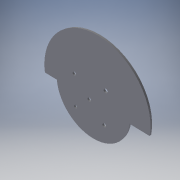
# Autodesk Inventor part: PanTilt_Base
Saved by Autodesk Inventor 2016 (Build 200138000, 138)
## iProperties
Created: 2016-04-18
Part Number: PanTilt_Base
Material: Generic
Document SubType Name: Modeling
Designer: Admin
Density: 1 g/cm^3
Appearance: Default
Author: Admin
Autodesk Inventor part; units mm, degrees
ref_plane "YZ Plane" through (0, 0, 0) normal (1, 0, 0) x (0, 1, 0)
ref_plane "XZ Plane" through (0, 0, 0) normal (0, 1, 0) x (-1, 0, 0)
ref_plane "XY Plane" through (0, 0, 0) normal (0, 0, 1) x (1, 0, 0)
sketch "Sketch1" plane through (0, 0, 0) normal (0, 1, 0) x (-1, 0, 0)
  line L0 (59.85, 0) -> (-59.85, 0) projected
  line L1 (0, -59.85) -> (0, 59.85) projected
  circle A0 centre (0, 0) radius 42.75
  line L2 (12.5, 12.5) -> (-12.5, 12.5) construction
  line L3 (-12.5, 12.5) -> (-12.5, -12.5) construction
  line L4 (-12.5, -12.5) -> (12.5, -12.5) construction
  line L5 (12.5, -12.5) -> (12.5, 12.5) construction
  circle A1 centre (12.5, 12.5) radius 1.5
  circle A2 centre (-12.5, 12.5) radius 1.5
  circle A3 centre (12.5, -12.5) radius 1.5
  circle A4 centre (-12.5, -12.5) radius 1.5
  circle A5 centre (0, 0) radius 1.5
  dimension "d0" = 85.5
  dimension "d1" = 25
  dimension "d2" = 25
  dimension "d3" = 12.5
  dimension "d4" = 12.5
  dimension "d5" = 3
  dimension "d8" = 25
  dimension "d11" = 25
  dimension "d16" = 3
  constraints: 8 end point, 6 centre point, 6 coincident, 2 horizontal, 2 parallel, 1 perpendicular, 1 vertical, 9 other
  measures "d0" diameter of A0
  measures "d1" distance of L2.start L2.end
  measures "d2" distance of L2.end L3.end
  measures "d3" distance between parallel lines of L0 L2
  measures "d4" distance between parallel lines of L1 L3
  measures "d5" diameter of A1
  measures "d8" distance of L2.start point (-12.5, 12.5)
  measures "d11" distance of L2.start point (12.5, -12.5)
  measures "d16" diameter of A5
extrude "Extrusion2" add sketch "Sketch1" along normal blind 1.4 contours A0 L1 A5 L0 | L0 A5 L1 A0 | L1 A5 L0 A0 | A0 L0 A5 L1
sketch "Sketch2" plane through (0, 1.4, 0) normal (0, 1, 0) x (1, 0, 0)
  circle A0 centre (0, 0) radius 1.5 projected
  arc A1 (30, 0) -> (-30, 0) centre (0, 0) ccw
  line L0 (-59.85, 0) -> (59.85, 0) projected
  line L1 (0, 59.85) -> (0, -59.85) projected
  arc A2 (42.75, 0) -> (-42.75, 0) centre (0, 0) ccw
  line L2 (-30, 0) -> (-42.75, 0)
  line L3 (30, 0) -> (42.75, 0)
  dimension "d19" = 60
  dimension "d20" = 85.5
  constraints: 4 end point, 4 point on circle, 4 point on line, 2 centre point, 2 coincident
  measures "d19" diameter of A1
  measures "d20" diameter of A2
extrude "Extrusion3" cut sketch "Sketch2" against normal blind 10 contours A1 L1 A2 L0 | A1 L0 A2 L1
equation "\"d2\" = d1"
equation "\"d3\" = 0.5 * d1"
equation "\"d4\" = 0.5 * d1"
body "Solid2"
